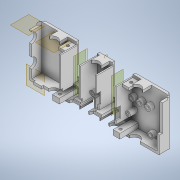
# Autodesk Inventor part: Part2
Saved by Autodesk Inventor 2022 (Build 260153000, 153)
## iProperties
Created: 2020-04-25
Part Number: Part2
Material: Generic
Document SubType Name: Modeling
Designer: Martijn
Density: 1 g/cm^3
Appearance: Default
Author: Martijn
Autodesk Inventor part; units mm, degrees
ref_plane "YZ Plane" through (0, 0, 0) normal (1, 0, 0) x (0, 1, 0)
ref_plane "XZ Plane" through (0, 0, 0) normal (0, 1, 0) x (-1, 0, 0)
ref_plane "XY Plane" through (0, 0, 0) normal (0, 0, 1) x (1, 0, 0)
sketch "Sketch1" plane through (0, 0, 0) normal (0, 0, 1) x (1, 0, 0)
  line L0 (0, 0) -> (0, 56)
  line L1 (0, 56) -> (41, 56)
  line L2 (41, 56) -> (41, 14)
  line L3 (41, 14) -> (66, 14)
  line L4 (66, 14) -> (66, 56)
  line L5 (66, 56) -> (84, 56)
  line L6 (84, 56) -> (84, 14)
  line L7 (84, 14) -> (109, 14)
  line L8 (109, 14) -> (109, 56)
  line L9 (109, 56) -> (150, 56)
  line L10 (150, 56) -> (150, 0)
  line L11 (150, 0) -> (0, 0)
  dimension "d0" = 150
  dimension "d1" = 41
  dimension "d2" = 41
  dimension "d3" = 56
  dimension "d4" = 25
  dimension "d5" = 25
  dimension "d6" = 14
  constraints: 24 end point, 8 perpendicular, 6 point on line, 1 vertical
  measures "d0" distance between parallel lines of L10 L0
  measures "d1" distance between parallel lines of L0 L2
  measures "d2" distance between parallel lines of L8 L10
  measures "d3" distance between parallel lines of L11 L1
  measures "d4" distance between parallel lines of L2 L4
  measures "d5" distance between parallel lines of L6 L8
  measures "d6" distance between parallel lines of L11 L3
extrude "Extrusion1" add sketch "Sketch1" along normal blind 3
sketch "Sketch2" plane through (0, 0, 0) normal (0, -1, 0) x (1, 0, 0)
  line L0 (0, 3) -> (-3, 6)
  line L1 (-3, 6) -> (-3, 3)
  line L2 (-3, 3) -> (0, 0)
  line L3 (0, 3) -> (150, 3) projected
  line L4 (0, 0) -> (0, 3) projected
  line L5 (150, 0) -> (150, 3) projected
  line L6 (150, 3) -> (153, 6)
  line L7 (153, 6) -> (153, 3)
  line L8 (153, 3) -> (150, 0)
  dimension "d9" = 135
  dimension "d10" = 3
  dimension "d11" = 3
  dimension "d12" = 135
  constraints: 12 end point, 3 parallel, 1 vertical
  measures "d9" angle of L3 L0
  measures "d10" distance between parallel lines of L4 L1
  measures "d11" distance between parallel lines of L5 L7
  measures "d12" angle of L3 L6
extrude "Extrusion2" add sketch "Sketch2" against normal up to surface (56 mm away)
sketch "Sketch3" plane through (0, 0, 0) normal (0, -1, 0) x (1, 0, 0)
  line L0 (0, 3) -> (-3, 6) projected
  line L1 (0, 3) -> (-3, 6)
  line L2 (153, 6) -> (150, 3) projected
  line L3 (-3, 15) -> (153, 15)
  line L4 (153, 6) -> (150, 3)
  line L5 (150, 3) -> (0, 3)
  line L6 (-3, 6) -> (-3, 15)
  line L7 (153, 6) -> (153, 15)
  line L8 (-3, 6) -> (-3, 3) projected
  line L9 (153, 3) -> (153, 6) projected
  point P0 (0, 0)
  dimension "d157" = 9
  constraints: 12 end point, 4 collinear, 1 horizontal, 1 parallel, 1 vertical
  measures "d157" distance of L3.end L4.start
extrude "Extrusion3" add sketch "Sketch3" against normal blind 3
sketch "Sketch4" plane through (0, 0, 0) normal (0, -1, 0) x (1, 0, 0)
  line L0 (-3, 15) -> (153, 15) projected
  line L1 (20.251, 15) -> (32.749, 15)
  line L2 (153, 15) -> (-3, 15) projected
  line L3 (20.251, 15) -> (20.251, 15)
  arc A0 (20.251, 15) -> (32.749, 15) centre (26.5, 15.8) ccw
  line L4 (0, 3) -> (150, 3) projected
  line L5 (0, 0) -> (150, 0) projected
  line L6 (-3, 15) -> (-3, 3) projected
  point P0 (139, 6)
  point P1 (32.749, 13)
  point P2 (20.251, 15)
  dimension "d24" = 6.3
  dimension "d155" = 12.8
  dimension "d175" = 29.5
  constraints: 4 end point, 2 point on circle, 1 centre point, 1 vertical, 5 other
  measures "d24" radius of A0
  measures "d155" distance from line of L4 A0.centre
  measures "d175" distance from line of L6 A0.centre
extrude "Extrusion4" cut sketch "Sketch4" against normal blind 3
pattern_linear "Rectangular Pattern1" count 5 spacing 24.25 along (1, 0, 0) of "Extrusion4"
sketch "Sketch6" plane through (153, 0, 3) normal (1, 0, 0) x (0, 0, -1)
  line L0 (0, 0) -> (0, 56) projected
  line L1 (0, 3) -> (0, 52.8)
  line L2 (0, 52.8) -> (-8.5, 52.8)
  line L3 (-8.5, 52.8) -> (-8.5, 21)
  line L4 (0, 56) -> (-3, 56) projected
  line L5 (-12, 3) -> (-12, 21)
  line L6 (-12, 21) -> (-8.5, 21)
  line L7 (-12, 3) -> (0, 3)
  line L8 (-12, 0) -> (-12, 3) projected
  point P0 (3, 0)
  point P1 (0, 3)
  dimension "d44" = 3.2
  dimension "d170" = 8.5
  dimension "d171" = 31.8
  constraints: 12 end point, 2 perpendicular, 2 point on line, 1 coincident, 1 collinear, 1 horizontal, 1 vertical
  measures "d44" distance between parallel lines of L4 L2
  measures "d170" distance between parallel lines of L0 L3
  measures "d171" distance between parallel lines of L2 L6
extrude "Extrusion6" add sketch "Sketch6" against normal blind 3
sketch "Sketch7" plane through (0, 0, 0) normal (0, -1, 0) x (1, 0, 0)
  line L0 (-3, 15) -> (153, 15) projected
  line L1 (4, 15) -> (13.6, 15)
  line L2 (13.6, 15) -> (13.6, 17)
  line L3 (13.6, 17) -> (4, 17)
  line L4 (4, 17) -> (4, 15)
  line L5 (-3, 15) -> (-3, 3) projected
  point P0 (0, 0)
  point P1 (139, 6)
  point P2 (13.6, 13)
  point P3 (153, 15)
  dimension "d46" = 9.6
  dimension "d47" = 2
  dimension "d160" = 7
  constraints: 8 end point, 2 parallel, 1 horizontal, 1 perpendicular, 2 other
  measures "d46" distance between parallel lines of L4 L2
  measures "d47" distance of L3.end L1.start
  measures "d160" distance between parallel lines of L5 L4
extrude "Extrusion7" add sketch "Sketch7" against normal blind 3
sketch "Sketch8" plane through (-3, 0, 3) normal (-1, 0, 0) x (0, 0, 1)
  arc A0 (12, 51.449) -> (12, 38.951) centre (12.8, 45.2) ccw
  line L0 (12, 3) -> (14, 3) projected
  line L1 (3, 56) -> (0, 56) projected
  arc A1 (12, 25.449) -> (12, 12.951) centre (12.8, 19.2) ccw
  line L2 (12, 38.951) -> (12, 25.449)
  line L3 (12, 0) -> (12, 3) projected
  line L4 (12, 12.951) -> (12, 3)
  line L5 (0, 56) -> (3, 56) projected
  line L6 (12, 52.8) -> (12, 51.449)
  line L7 (10, 3) -> (10, 0) projected
  line L8 (3, 3) -> (14, 3) projected
  line L9 (0, 3) -> (12, 3)
  line L10 (-3, 56) -> (0, 56) projected
  line L11 (12, 52.8) -> (0, 52.8)
  line L12 (0, 0) -> (0, 56) projected
  line L13 (0, 52.8) -> (0, 3)
  point P0 (-3, 0)
  dimension "d51" = 6.3
  dimension "d159" = 6.3
  dimension "d161" = 26
  dimension "d179" = 3.2
  dimension "d180" = 10.8
  dimension "d181" = 12.8
  dimension "d182" = 12.8
  constraints: 12 end point, 5 point on circle, 3 collinear, 2 centre point, 2 vertical, 1 point on line, 1 other
  measures "d51" radius of A0
  measures "d159" radius of A1
  measures "d161" distance of A0.centre A1.centre
  measures "d179" distance between parallel lines of L11 L1
  measures "d180" distance from line of L5 A0.centre
  measures "d181" distance from line of L12 A0.centre
  measures "d182" distance from line of L12 A1.centre
extrude "Extrusion8" add sketch "Sketch8" against normal blind 3
sketch "Sketch9" plane through (109, 56, 3) normal (0, 1, 0) x (1, 0, 0)
  line L0 (-68, 0) -> (-109, 0) projected
  line L1 (-77.9, 0) -> (-90.1, 0)
  arc A0 (-78.3564, -10) -> (-89.6436, -10) centre (-84, -12.8) ccw
  line L2 (-109, 0) -> (-109, -12) projected
  line L3 (-78.3564, -10) -> (-77.9, -10)
  line L4 (-77.9, -10) -> (-77.9, 0)
  line L5 (-89.6436, -10) -> (-90.1, -10)
  line L6 (-90.1, -10) -> (-90.1, 0)
  point P0 (-109, 3)
  dimension "d63" = 6.3
  dimension "d64" = 12.8
  dimension "d183" = 25
  dimension "d186" = 10
  dimension "d187" = 12.2
  constraints: 10 end point, 2 collinear, 2 horizontal, 2 perpendicular, 2 point on circle, 2 point on line, 1 centre point
  measures "d63" radius of A0
  measures "d64" distance from line of L1 A0.centre
  measures "d183" distance from line of L2 A0.centre
  measures "d186" distance between parallel lines of L0 L3
  measures "d187" distance between parallel lines of L4 L6
extrude "Extrusion9" add sketch "Sketch9" against normal blind 3.2
pattern_linear "Rectangular Pattern3" count 3 spacing 50 along (1, 0, 0) of "Extrusion9"
sketch "Sketch18" plane through (0, 0, 3) normal (0, 0, 1) x (1, 0, 0)
  line L0 (0, 3) -> (150, 3) projected
  line L1 (34.625, 3) -> (42.625, 3)
  line L2 (42.625, 3) -> (42.625, 9)
  line L3 (42.625, 9) -> (34.625, 9)
  line L4 (34.625, 9) -> (34.625, 3)
  line L5 (0, 3) -> (150, 3) projected
  line L6 (32.749, 3) -> (68.751, 3) projected
  line L7 (115.4, 9) -> (107.4, 9)
  line L8 (107.4, 9) -> (107.4, 3)
  line L9 (107.4, 3) -> (115.4, 3)
  line L10 (115.4, 3) -> (115.4, 9)
  line L11 (153, 0) -> (153, 56) projected
  line L12 (-3, 0) -> (-3, 12.951) projected
  point P0 (0, 0)
  point P1 (39.5, 3)
  point P2 (42.625, 3)
  point P3 (44.65, 3)
  point P4 (55.5, 3)
  point P5 (94.5, 3)
  point P6 (108.4, 3)
  point P7 (4, 3)
  point P8 (110.5, 3)
  dimension "d126" = 6
  dimension "d138" = 6
  dimension "d163" = 8
  dimension "d190" = 37.6
  dimension "d191" = 37.625
  dimension "d192" = 8
  constraints: 16 end point, 4 parallel, 2 horizontal, 2 perpendicular, 1 coincident, 1 collinear, 1 point on line
  measures "d126" distance between parallel lines of L0 L3
  measures "d138" distance between parallel lines of L9 L7
  measures "d163" distance between parallel lines of L2 L4
  measures "d190" distance between parallel lines of L10 L11
  measures "d191" distance between parallel lines of L12 L4
  measures "d192" distance between parallel lines of L10 L8
extrude "Extrusion16" add sketch "Sketch18" along normal blind 22
sketch "Sketch19" plane through (34.625, 3, 15) normal (0, -1, 0) x (1, 0, 0)
  circle A0 centre (4, 5.2) radius 1.6
  line L0 (0, 10) -> (8, 10) projected
  circle A1 centre (76.775, 5.2) radius 1.6
  line L1 (80.775, -12) -> (115.375, -12) projected
  line L2 (72.775, 0) -> (72.775, 10) projected
  line L3 (8, 0) -> (8, 10) projected
  line L4 (72.775, 10) -> (80.775, 10) projected
  point P0 (-34.625, -15)
  point P1 (8, 10)
  dimension "d131" = 3.2
  dimension "d132" = 4.8
  dimension "d139" = 3.2
  dimension "d162" = 4
  dimension "d262" = 4
  dimension "d263" = 4.8
  constraints: 2 centre point
  measures "d131" diameter of A0
  measures "d132" distance from line of L0 A0.centre
  measures "d139" diameter of A1
  measures "d162" distance from line of L2 A1.centre
  measures "d262" distance from line of L3 A0.centre
  measures "d263" distance from line of L4 A1.centre
extrude "Extrusion17" cut sketch "Sketch19" against normal blind 10
ref_plane "Work Plane2" through (-8, 52.8, 11) normal (0, 1, 0) x (1, 0, 0)
sketch "Sketch20" plane through (-8, 52.8, 11) normal (0, 1, 0) x (1, 0, 0)
  circle A0 centre (20, 4) radius 1.6
  line L0 (39.1, 8) -> (26.9, 8) projected
  line L1 (5, 8) -> (5, 5) projected
  circle A1 centre (146, 4) radius 1.6
  line L2 (161, 5) -> (161, -0.5) projected
  line L3 (139.1, 8) -> (158, 8) projected
  point P0 (8, 11)
  point P1 (8, 8)
  dimension "d142" = 4
  dimension "d143" = 3.2
  dimension "d144" = 15
  dimension "d145" = 3.2
  dimension "d184" = 15
  dimension "d185" = 4
  constraints: 2 centre point
  measures "d142" distance from line of L0 A0.centre
  measures "d143" diameter of A0
  measures "d144" distance from line of L1 A0.centre
  measures "d145" diameter of A1
  measures "d184" distance from line of L2 A1.centre
  measures "d185" distance from line of L3 A1.centre
extrude "Extrusion18" cut sketch "Sketch20" against normal blind 10
ref_plane "Work Plane4" through (0, 0, 11) normal (0, 0, 1) x (1, 0, 0)
ref_plane "Work Plane3" through (25, 52.8, 13.8) normal (0, 1, 0) x (1, 0, 0)
sketch "Sketch23" plane through (25, 52.8, 13.8) normal (0, 1, 0) x (1, 0, 0)
  circle A0 centre (0, 0) radius 6.3
  arc A1 (5.6436, 2.8) -> (-5.6436, 2.8) centre (0, 0) ccw projected
  point P0 (-25, 13.8)
  constraints: 2 concentric, 1 centre point
extrude "Extrusion21" cut sketch "Sketch23" against normal blind 10
sketch "Sketch24" plane through (0, 0, 0) normal (0, 0, -1) x (-1, 0, 0)
  line L0 (0, 0) -> (-150, 0) projected
  line L1 (-58.124, 0) -> (-67.624, 0)
  line L2 (-67.624, 0) -> (-67.624, 12.5)
  line L3 (-67.624, 12.5) -> (-58.124, 12.5)
  line L4 (-58.124, 12.5) -> (-58.124, 0)
  line L5 (-82.374, 0) -> (-91.874, 0)
  line L6 (-91.874, 0) -> (-91.874, 12.5)
  line L7 (-91.874, 12.5) -> (-82.374, 12.5)
  line L8 (-82.374, 12.5) -> (-82.374, 0)
  line L9 (-68.751, 0) -> (-68.751, 3) projected
  line L10 (-56.999, 3) -> (-56.999, 0) projected
  line L11 (-81.249, 3) -> (-81.249, 0) projected
  point P0 (-62.874, 0)
  point P1 (-87.124, 0)
  point P2 (-91.874, 0)
  point P3 (-82.374, 0)
  point P4 (-67.624, 0)
  dimension "d196" = 9.5
  dimension "d197" = 9.5
  dimension "d198" = 11.752
  dimension "d199" = 5.875
  dimension "d200" = 5.875
  dimension "d201" = 12.5
  dimension "d202" = 12.5
  constraints: 16 end point, 4 parallel, 2 horizontal, 2 midpoint, 2 perpendicular, 2 point on line
  measures "d196" distance between parallel lines of L4 L2
  measures "d197" distance between parallel lines of L6 L8
  measures "d198" distance between parallel lines of L9 L10
  measures "d199" distance from line of L10 point (-62.874, 0)
  measures "d200" distance from line of point (-87.124, 0) L11
  measures "d201" distance between parallel lines of L0 L7
  measures "d202" distance between parallel lines of L3 L0
extrude "Extrusion22" cut sketch "Sketch24" against normal blind 30
sketch "Sketch25" plane through (0, 0, 3) normal (0, 0, 1) x (1, 0, 0)
  line L0 (67.624, 3) -> (68.751, 3) projected
  line L1 (67.624, 3) -> (69.124, 3)
  line L2 (69.124, 3) -> (69.124, 14)
  line L3 (69.124, 14) -> (56.624, 14)
  line L4 (56.624, 14) -> (56.624, 3)
  line L5 (115.4, 3) -> (58.124, 3) projected
  line L6 (67.624, 12.5) -> (58.124, 12.5) projected
  line L7 (58.124, 3) -> (58.124, 12.5)
  line L8 (58.124, 12.5) -> (67.624, 12.5)
  line L9 (67.624, 12.5) -> (67.624, 3) projected
  line L10 (67.624, 12.5) -> (67.624, 3)
  line L11 (42.625, 3) -> (58.124, 3) projected
  line L12 (58.124, 3) -> (56.624, 3)
  point P0 (0, 0)
  point P1 (67.624, 3)
  point P2 (67.624, 3)
  point P3 (69.124, 3)
  dimension "d205" = 1.5
  dimension "d206" = 1.5
  dimension "d207" = 1.5
  constraints: 16 end point, 4 perpendicular, 2 vertical, 1 collinear, 1 point on line
  measures "d205" distance between parallel lines of L2 L9
  measures "d206" distance between parallel lines of L7 L4
  measures "d207" distance between parallel lines of L6 L3
extrude "Extrusion23" add sketch "Sketch25" along normal blind 5 contours L9 L6 L7 L11 L4 L3 L2 L1 L0
sketch "Sketch26" plane through (0, 0, 3) normal (0, 0, 1) x (1, 0, 0)
  line L0 (41, 14) -> (66, 14)
  line L1 (64.5, 15.5) -> (42.5, 15.5)
  line L2 (41, 14) -> (41, 56) projected
  line L3 (64.5, 15.5) -> (64.5, 53)
  line L4 (64.5, 53) -> (66, 53)
  line L5 (66, 14) -> (41, 14) projected
  line L6 (66, 14) -> (66, 53)
  line L7 (66, 56) -> (66, 14) projected
  line L8 (68.9, 56) -> (66, 56) projected
  line L9 (42.5, 15.5) -> (42.5, 53)
  line L10 (42.5, 53) -> (41, 53)
  line L11 (41, 14) -> (41, 56) projected
  line L12 (41, 14.5075) -> (41, 53)
  line L13 (41, 56) -> (31.1, 56) projected
  point P0 (0, 0)
  dimension "d212" = 1.5
  dimension "d239" = 1.5
  dimension "d240" = 3
  dimension "d241" = 1.5
  dimension "d242" = 3
  constraints: 16 end point, 2 collinear, 2 perpendicular, 2 point on line, 2 vertical
  measures "d212" distance between parallel lines of L0 L1
  measures "d239" distance between parallel lines of L6 L3
  measures "d240" distance between parallel lines of L8 L4
  measures "d241" distance between parallel lines of L2 L9
  measures "d242" distance between parallel lines of L13 L10
extrude "Extrusion24" add sketch "Sketch26" along normal blind 5 and the other way blind 1.5
sketch "Sketch27" plane through (0, 0, 8) normal (0, 0, 1) x (1, 0, 0)
  line L0 (41, 14) -> (66, 14) projected
  line L1 (41, 53) -> (42.5, 53)
  line L2 (42.5, 53) -> (42.5, 14)
  line L3 (42.5, 14) -> (41, 14)
  line L4 (41, 14) -> (41, 53)
  line L5 (64.5, 15.5) -> (42.5, 15.5) projected
  line L6 (58.124, 15.5) -> (58.124, 14)
  line L7 (41, 14) -> (66, 14) projected
  line L8 (64.5, 15.5) -> (58.124, 15.5)
  line L9 (56.624, 14) -> (56.624, 3) projected
  line L10 (58.124, 3) -> (58.124, 12.5) projected
  line L11 (42.5, 53) -> (41, 53) projected
  line L12 (66, 53) -> (64.5, 53) projected
  line L13 (66, 14) -> (66, 53)
  line L14 (66, 53) -> (64.5, 53)
  line L15 (64.5, 53) -> (64.5, 15.5) projected
  line L16 (64.5, 53) -> (64.5, 15.5)
  line L17 (42.5, 15.5) -> (42.5, 53) projected
  line L18 (41, 53) -> (41, 14) projected
  point P0 (0, 0)
  point P1 (66, 56)
  constraints: 18 end point, 4 collinear, 3 equal length, 3 perpendicular, 3 point on line, 1 horizontal, 1 vertical
extrude "Extrusion25" add sketch "Sketch27" along normal blind 10 contours L4 L1 L2 L0 | L6 L5 L15 L12 L13 L0
sketch "Sketch28" plane through (0, 0, 8) normal (0, 0, 1) x (1, 0, 0)
  line L0 (58.124, 14) -> (67.624, 14)
  line L1 (67.624, 14) -> (67.624, 12.5)
  line L2 (67.624, 12.5) -> (58.124, 12.5)
  line L3 (58.124, 12.5) -> (58.124, 14)
  line L4 (58.124, 3) -> (58.124, 12.5) projected
  line L5 (66, 14) -> (58.124, 14) projected
  point P0 (0, 0)
  constraints: 8 end point, 2 collinear, 2 parallel, 1 horizontal, 1 perpendicular
extrude "Extrusion26" add sketch "Sketch28" along normal blind 16
chamfer "Chamfer6" distance 1.5 angle 45 3 edges at (53.5, 15.5, 1.5) (42.5, 34.25, 1.5) (64.5, 34.25, 1.5)
sketch "Sketch29" plane through (0, 0, 0) normal (0, 0, -1) x (-1, 0, 0)
  line L0 (-48, 18) -> (-38, 18)
  arc A0 (-38, 18) -> (-35, 21) centre (-38, 21) ccw
  line L1 (-35, 21) -> (-35, 31)
  arc A1 (-35, 31) -> (-48, 18) centre (-38, 21) ccw
  line L2 (0, 56) -> (0, 0) projected
  line L3 (-41, 14) -> (-41, 56) projected
  line L4 (0, 3) -> (-34.625, 3) projected
  dimension "d224" = 3
  dimension "d225" = 6
  dimension "d226" = 90
  dimension "d227" = 10
  dimension "d230" = 18
  constraints: 4 end point, 4 point on circle, 2 centre point, 2 tangent, 1 coincident, 1 parallel
  measures "d224" radius of A0
  measures "d225" distance between parallel lines of L3 L1
  measures "d226" angle of L1 L0
  measures "d227" distance of L1.start L1.end
  measures "d230" distance from line of L4 A0.centre
extrude "Extrusion27" cut sketch "Sketch29" against normal blind 2
sketch "Sketch30" plane through (0, 0, 2) normal (0, 0, -1) x (-1, 0, 0)
  arc A0 (-38, 18) -> (-35, 21) centre (-38, 21) ccw projected
  circle A1 centre (-38, 21) radius 3
  point P0 (0, 0)
  point P1 (-38, 18)
  dimension "d231" = 6
  constraints: 1 centre point, 1 coincident
  measures "d231" diameter of A1
extrude "Extrusion28" add sketch "Sketch30" against normal blind 10
sketch "Sketch31" plane through (0, 0, 2) normal (0, 0, -1) x (-1, 0, 0)
  circle A0 centre (-38, 21) radius 1.25
  arc A1 (-38, 18) -> (-35, 21) centre (-38, 21) ccw projected
  point P0 (0, 0)
  dimension "d234" = 2.5
  constraints: 1 centre point, 1 concentric
  measures "d234" diameter of A0
extrude "Extrusion29" cut sketch "Sketch31" against normal blind 10
ref_plane "Work Plane7" through (53.5, 15.5, 18) normal (-1, 0, 0) x (0, 0, 1)
mirror "Mirror5" about plane through (53.5, 15.5, 18) normal (-1, 0, 0) of "Extrusion28", "Extrusion27", "Extrusion29"
ref_plane "Work Plane6" through (75, 14, 0) normal (1, 0, 0) x (0, 0, -1)
mirror "Mirror4" about plane through (75, 14, 0) normal (1, 0, 0) of "Extrusion27", "Extrusion28", "Extrusion29", "Extrusion23", "Extrusion26", "Extrusion25", "Extrusion24", "Chamfer6", "Mirror5"
sketch "Sketch32" plane through (0, 0, 3) normal (0, 0, 1) x (1, 0, 0)
  line L0 (117.2, 52.8) -> (109, 52.8)
  line L1 (109, 52.8) -> (109, 49.8)
  line L2 (109, 49.8) -> (117.2, 49.8)
  line L3 (117.2, 49.8) -> (117.2, 52.8)
  line L4 (150, 56) -> (131.1, 56) projected
  line L5 (109, 53) -> (109, 21) projected
  line L6 (118.9, 52.8) -> (118.9, 56) projected
  line L7 (131.1, 56) -> (131.1, 52.8) projected
  line L8 (41, 53) -> (42.5, 53) projected
  line L9 (41.0301, 52.8) -> (32.8, 52.8)
  line L10 (32.8, 52.8) -> (32.8, 49.8)
  line L11 (32.8, 49.8) -> (41.0301, 49.8)
  line L12 (41.0301, 49.8) -> (41.0301, 52.8)
  line L13 (31.1, 56) -> (31.1, 52.8) projected
  line L14 (41, 56) -> (31.1, 56) projected
  point P0 (0, 0)
  dimension "d244" = 3.2
  dimension "d245" = 3
  dimension "d246" = 12.2
  dimension "d247" = 1.7
  dimension "d253" = 1.7
  dimension "d260" = 3.2
  constraints: 16 end point, 4 parallel, 2 collinear, 2 horizontal, 2 perpendicular
  measures "d244" distance between parallel lines of L4 L0
  measures "d245" distance between parallel lines of L0 L2
  measures "d246" distance between parallel lines of L6 L7
  measures "d247" distance between parallel lines of L6 L3
  measures "d253" distance between parallel lines of L13 L10
  measures "d260" distance between parallel lines of L14 L9
extrude "Extrusion30" add sketch "Sketch32" along normal blind 13
sketch "Sketch33" plane through (109, 52.8, 3) normal (0, 1, 0) x (1, 0, 0)
  circle A0 centre (4, -6) radius 1.6
  line L0 (44, 0) -> (44, -3) projected
  line L1 (0, 0) -> (8.2, 0) projected
  circle A1 centre (-72, -6) radius 1.6
  line L2 (-76.2, 0) -> (-68, 0) projected
  point P0 (-109, 3)
  point P1 (-112, -3)
  dimension "d250" = 40
  dimension "d255" = 3.2
  dimension "d256" = 6
  dimension "d257" = 3.2
  dimension "d259" = 40
  dimension "d261" = 6
  constraints: 2 centre point
  measures "d250" distance from line of L0 A0.centre
  measures "d255" diameter of A0
  measures "d256" distance from line of A0.centre L1
  measures "d257" diameter of A1
  measures "d259" horizontal distance of point (-112, -3) A1.centre
  measures "d261" distance from line of A1.centre L2
extrude "Extrusion31" cut sketch "Sketch33" against normal blind 10
sketch "Sketch34" plane through (0, 0, 3) normal (0, 0, 1) x (1, 0, 0)
  circle A0 centre (134.749, 8) radius 2
  circle A1 centre (131.5, 35) radius 2
  circle A2 centre (121.5, 35) radius 2
  circle A3 centre (111.5, 35) radius 2
  line L0 (115.4, 3) -> (150, 3) projected
  line L1 (129.749, 3) -> (129.749, 0) projected
  circle A4 centre (81.5, 34) radius 2
  line L2 (68.751, 3) -> (81.249, 3) projected
  line L3 (84, 21) -> (84, 53) projected
  line L4 (109, 49.8) -> (109, 21) projected
  circle A5 centre (34.749, 16) radius 2
  line L5 (0, 3) -> (34.625, 3) projected
  line L6 (32.749, 3) -> (32.749, 0) projected
  point P0 (0, 0)
  dimension "d264" = 4
  dimension "d265" = 32
  dimension "d266" = 32
  dimension "d267" = 32
  dimension "d268" = 4
  dimension "d269" = 4
  dimension "d270" = 4
  dimension "d271" = 5
  dimension "d274" = 10
  dimension "d275" = 10
  dimension "d276" = 5
  dimension "d277" = 31
  dimension "d278" = 4
  dimension "d279" = 2.5
  dimension "d280" = 2.5
  dimension "d281" = 4
  dimension "d282" = 13
  dimension "d283" = 2
  constraints: 6 centre point
  measures "d264" diameter of A3
  measures "d265" distance from line of L0 A3.centre
  measures "d266" distance from line of L0 A2.centre
  measures "d267" distance from line of L0 A1.centre
  measures "d268" diameter of A2
  measures "d269" diameter of A1
  measures "d270" diameter of A0
  measures "d271" distance from line of L0 A0.centre
  measures "d274" distance of A2.centre A3.centre
  measures "d275" distance of A1.centre A2.centre
  measures "d276" distance from line of A0.centre L1
  measures "d277" distance from line of L2 A4.centre
  measures "d278" diameter of A4
  measures "d279" distance from line of L3 A4.centre
  measures "d280" distance from line of L4 A3.centre
  measures "d281" diameter of A5
  measures "d282" distance from line of L5 A5.centre
  measures "d283" distance from line of L6 A5.centre
extrude "Extrusion32" cut sketch "Sketch34" against normal blind 2.7
sketch "Sketch36" plane through (0, 0, 18) normal (0, 0, 1) x (1, 0, 0)
  line L0 (42.5, 53) -> (41, 53) projected
  line L1 (41, 14) -> (42.5, 14) projected
  line L2 (42.5, 53) -> (41, 53)
  line L3 (41, 53) -> (41, 14)
  line L4 (41, 14) -> (42.5, 14)
  line L5 (42.5, 14) -> (42.5, 53)
  line L6 (64.5, 53) -> (64.5, 15.5) projected
  line L7 (64.5, 53) -> (66, 53)
  line L8 (58.124, 14) -> (66, 14) projected
  line L9 (66, 53) -> (66, 14)
  line L10 (66, 14) -> (58.124, 14)
  line L11 (58.124, 14) -> (58.124, 15.5)
  line L12 (58.124, 15.5) -> (64.5, 15.5)
  line L13 (66, 53) -> (64.5, 53) projected
  line L14 (64.5, 15.5) -> (64.5, 53)
  line L15 (58.124, 15.5) -> (58.124, 14) projected
  line L16 (84, 53) -> (85.5, 53) projected
  line L17 (85.5, 53) -> (85.5, 15.5) projected
  line L18 (84, 53) -> (85.5, 53)
  line L19 (85.5, 53) -> (85.5, 34)
  line L20 (85.5, 34) -> (84, 34)
  line L21 (84, 34) -> (84, 53)
  line L22 (84, 14) -> (84, 53) projected
  line L23 (84, 21) -> (85.5, 21)
  line L24 (85.5, 15.5) -> (91.876, 15.5) projected
  line L25 (85.5, 15.5) -> (91.876, 15.5)
  line L26 (91.876, 14) -> (84, 14) projected
  line L27 (91.876, 15.5) -> (91.876, 14)
  line L28 (91.876, 14) -> (84, 14)
  line L29 (84, 14) -> (84, 21)
  line L30 (107.5, 53) -> (109, 53)
  line L31 (109, 53) -> (109, 31)
  line L32 (109, 31) -> (107.5, 31)
  line L33 (107.5, 31) -> (107.5, 53)
  line L34 (109, 53) -> (109, 14) projected
  line L35 (107.5, 14) -> (109, 14)
  line L36 (109, 14) -> (109, 18)
  line L37 (109, 18) -> (107.5, 18)
  line L38 (107.5, 18) -> (107.5, 14)
  point P0 (0, 0)
  point P1 (109, 49.8)
  point P2 (109, 14)
  dimension "d288" = 19
  dimension "d289" = 13
  dimension "d290" = 22
  dimension "d291" = 13
  constraints: 54 end point, 11 perpendicular, 10 equal length, 6 horizontal, 4 point on line, 2 collinear
  measures "d288" distance of L20.end L16.start
  measures "d289" distance between parallel lines of L23 L20
  measures "d290" distance between parallel lines of L30 L32
  measures "d291" distance between parallel lines of L37 L32
extrude "Extrusion33" add sketch "Sketch36" along normal blind 5 contours L5 L1 L3 L0 | L7 L9 L8 L11 L12 L6 | L16 L17 L20 L21 | L23 L17 L24 L27 L26 L22 | L30 L31 L32 L33 | L34 L35 L38 L37
fillet "Fillet2" radius 1 12 edges at (153, 56, 4.5) (151.5, 56, 1.5) (151.5, 0, 1.5) (153, 0, 9) (-3, 0, 9) (-1.5, 0, 1.5) (-3, 56, 4.5) (-1.5, 56, 1.5) (91.874, 0, 7.5) (82.374, 0, 7.5) (67.624, 0, 7.5) (58.124, 0, 7.5)
sketch "Sketch37" plane through (0, 0, 3) normal (0, 0, 1) x (1, 0, 0)
  circle A0 centre (111.5, 35) radius 3.5
  circle A1 centre (121.5, 35) radius 3.5
  circle A2 centre (131.5, 35) radius 2 projected
  circle A3 centre (131.5, 35) radius 3.5
  circle A4 centre (111.5, 35) radius 2 projected
  circle A5 centre (121.5, 35) radius 2 projected
  point P0 (0, 0)
  dimension "d293" = 1.5
  dimension "d294" = 1.5
  dimension "d295" = 1.5
  constraints: 3 centre point, 2 concentric, 1 coincident
  measures "d293" radial gap between concentric circles of A3 A2
  measures "d294" radial gap between concentric circles of A1 A5
  measures "d295" radial gap between concentric circles of A4 A0
extrude "Extrusion34" add sketch "Sketch37" along normal blind 5
sketch "Sketch38" plane through (0, 0, 3) normal (0, 0, 1) x (1, 0, 0)
  circle A0 centre (34.749, 16) radius 3.5
  circle A1 centre (34.749, 16) radius 2 projected
  circle A2 centre (81.5, 34) radius 3.5
  circle A3 centre (81.5, 34) radius 2 projected
  circle A4 centre (134.749, 8) radius 3.5
  circle A5 centre (134.749, 8) radius 2
  circle A6 centre (134.749, 8) radius 2 projected
  point P0 (0, 0)
  dimension "d298" = 1.5
  dimension "d309" = 1.5
  dimension "d310" = 1.5
  constraints: 4 centre point, 4 concentric, 1 coincident
  measures "d298" radial gap between concentric circles of A0 A1
  measures "d309" radial gap between concentric circles of A2 A3
  measures "d310" radial gap between concentric circles of A5 A4
extrude "Extrusion35" add sketch "Sketch38" along normal blind 5
sketch "Sketch39" plane through (0, 0, 23) normal (0, 0, 1) x (1, 0, 0)
  line L0 (64.5, 53) -> (64.5, 15.5) projected
  line L1 (66, 14) -> (66, 53) projected
  line L2 (64.5, 15.5) -> (66, 15.5)
  line L3 (66, 15.5) -> (66, 18.5)
  line L4 (66, 18.5) -> (64.5, 18.5)
  line L5 (64.5, 18.5) -> (64.5, 15.5)
  point P0 (0, 0)
  dimension "d301" = 3
  constraints: 8 end point, 2 parallel, 1 horizontal, 1 perpendicular, 1 point on line
  measures "d301" distance between parallel lines of L2 L4
extrude "Extrusion36" cut sketch "Sketch39" against normal blind 2.5
sketch "Sketch40" plane through (0, 0, 23) normal (0, 0, 1) x (1, 0, 0)
  line L0 (42.5, 14) -> (42.5, 53) projected
  line L1 (41, 14) -> (42.5, 14)
  line L2 (42.5, 14) -> (42.5, 17)
  line L3 (42.5, 17) -> (41, 17)
  line L4 (41, 17) -> (41, 14)
  point P0 (0, 0)
  dimension "d304" = 3
  constraints: 8 end point, 2 parallel, 1 horizontal, 1 perpendicular, 1 point on line
  measures "d304" distance between parallel lines of L1 L3
extrude "Extrusion37" cut sketch "Sketch40" against normal blind 2.5
sketch "Sketch41" plane through (0, 0, 23) normal (0, 0, 1) x (1, 0, 0)
  line L0 (85.5, 15.5) -> (85.5, 21) projected
  line L1 (84, 21) -> (85.5, 21)
  line L2 (85.5, 21) -> (85.5, 15.5)
  line L3 (85.5, 15.5) -> (84, 15.5)
  line L4 (84, 15.5) -> (84, 21)
  point P0 (0, 0)
  constraints: 8 end point, 2 parallel, 1 horizontal, 1 perpendicular
extrude "Extrusion38" cut sketch "Sketch41" against normal blind 3
ref_plane "Work Plane8" through (53.5, 15.5, 18) normal (-1, 0, 0) x (0, 0, 1)
ref_plane "Work Plane9" through (96.5, 15.5, 18) normal (-1, 0, 0) x (0, 0, 1)
ref_plane "Work Plane10" through (96.5, 15.5, 18) normal (-1, 0, 0) x (0, 0, 1)
body "Solid1"
